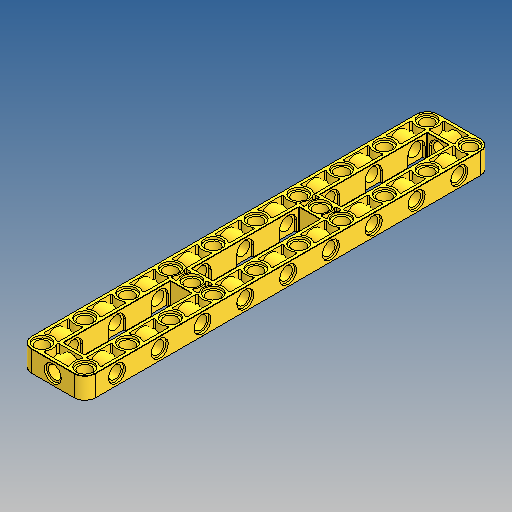
# Autodesk Inventor part: 67491-Yellow
Saved by Autodesk Inventor 2025 (Build 290162010, 162A)
## iProperties
Created: 2012-03-21
Part Number: 67491-Yellow
Document SubType Name: Modeling
Designer: h.muther
Density: 1.06 g/cm^3
Material: ABS Plastic
Mass: 5.69641 g
Surface Area: 80.0064 cm^2
Volume: 5.37397 cm^3
Appearance: Yellow
Author: h.muther
Autodesk Inventor part; units mm, degrees
ref_plane "YZ Plane" through (0, 0, 0) normal (1, 0, 0) x (0, 1, 0)
ref_plane "XZ Plane" through (0, 0, 0) normal (0, 1, 0) x (-1, 0, 0)
ref_plane "XY Plane" through (0, 0, 0) normal (0, 0, 1) x (1, 0, 0)
sketch "Sketch1" plane through (0, 0, 0) normal (0, 0, 1) x (1, 0, 0)
  line L0 (4, -24) -> (4, 24)
  line L1 (-4, 24) -> (-4, -24)
  arc A0 (4, 24) -> (2.8284, 26.8284) centre (0, 24) ccw construction
  arc A1 (-4, -24) -> (4, -24) centre (0, -24) ccw
  circle A2 centre (0, 24) radius 3.2
  circle A3 centre (0, 24) radius 2.4
  line L2 (2.8284, 21.1716) -> (2.8284, 10.8284)
  line L3 (-2.8284, 21.1716) -> (-2.8284, 10.8284)
  arc A4 (-2.8284, 21.1716) -> (2.8284, 21.1716) centre (0, 24) ccw
  arc A5 (2.8284, 10.8284) -> (-2.8284, 10.8284) centre (0, 8) ccw
  circle A6 centre (0, 8) radius 3.2
  circle A7 centre (0, 8) radius 2.4
  line L4 (2.8284, 5.1716) -> (2.8284, -5.1716)
  line L5 (-2.8284, 5.1716) -> (-2.8284, -5.1716)
  arc A8 (-2.8284, 5.1716) -> (2.8284, 5.1716) centre (0, 8) ccw
  arc A9 (2.8284, -5.1716) -> (-2.8284, -5.1716) centre (0, -8) ccw
  circle A10 centre (0, -8) radius 3.2
  circle A11 centre (0, -8) radius 2.4
  line L6 (2.8284, -10.8284) -> (2.8284, -21.1716)
  line L7 (-2.8284, -10.8284) -> (-2.8284, -21.1716)
  arc A12 (-2.8284, -10.8284) -> (2.8284, -10.8284) centre (0, -8) ccw
  arc A13 (2.8284, -21.1716) -> (-2.8284, -21.1716) centre (0, -24) ccw
  circle A14 centre (0, -24) radius 3.2
  circle A15 centre (0, -24) radius 2.4
  line L8 (0, 24) -> (-2.8284, 21.1716) construction
  line L9 (-4, 24) -> (-4, 40)
  line L10 (4, 40) -> (4, 24)
  arc A16 (-2.4, 40) -> (2.4, 40) centre (0, 40) ccw
  arc A17 (-3.2, 40) -> (3.2, 40) centre (0, 40) ccw
  line L11 (-4, 40) -> (-2.4, 40)
  line L12 (2.4, 40) -> (4, 40)
  line L13 (-2.8284, 37.1716) -> (-2.8284, 26.8284)
  arc A18 (2.8284, 26.8284) -> (-2.8284, 26.8284) centre (0, 24) ccw
  arc A19 (-2.8284, 37.1716) -> (2.8284, 37.1716) centre (0, 40) ccw
  line L14 (2.8284, 37.1716) -> (2.8284, 26.8284)
  arc A20 (-2.8284, 26.8284) -> (-4, 24) centre (0, 24) ccw construction
  arc A21 (2.8284, 26.8284) -> (-2.8284, 26.8284) centre (0, 24) ccw
  arc A22 (2.4, 40) -> (-2.4, 40) centre (0, 40) ccw
  arc A23 (3.2, 40) -> (-3.2, 40) centre (0, 40) ccw
  line L15 (-4, 40) -> (-4, 48)
  line L16 (-4, 48) -> (4, 48)
  line L17 (4, 48) -> (4, 40)
  line L18 (-2.8284, 48) -> (-2.8284, 42.8284)
  line L19 (2.8284, 48) -> (2.8284, 42.8284)
  arc A24 (2.8284, 42.8284) -> (-2.8284, 42.8284) centre (0, 40) ccw
  point P0 (0, 0)
  point P1 (-4, 0)
  dimension "d48" = 48
  dimension "d49" = 6.4
  dimension "d50" = 4.8
  dimension "d51" = 16
  dimension "d64" = 16
  dimension "d116" = 45
  dimension "d117" = 56
  dimension "d118" = 8
  dimension "d119" = 16
  dimension "d134" = 8
  constraints: 40 end point, 34 point on circle, 25 centre point, 10 coincident, 9 equal radius, 9 tangent, 7 collinear, 7 vertical, 5 perpendicular, 3 concentric, 3 horizontal alignment, 3 midpoint, 3 point on line, 2 parallel, 2 vertical alignment, 28 other
  measures "d48" distance of A1.centre A0.centre
  measures "d49" diameter of A2
  measures "d50" diameter of A3
  measures "d51" distance of A0.centre A5.centre
  measures "d64" distance of L3.start L5.start
  measures "d116" angle of L8 L1
  measures "d118" diameter of A0
  measures "d119" distance of A16.centre A3.centre
  measures "d134" distance from line of A23.centre L16
extrude "Extrusion1" add sketch "Sketch1" along normal mid plane 8 contours A1 L1 L9 L11 A17 L12 L10 L0 | L12 A23 L11 L15 L16 L18 A24 L19 L17 | A17 L11 A16 L12 | L12 A22 L11 A23 | L19 A24 L18 L16 | A2 | L2 A5 L3 A4 | A6 | L4 A9 L5 A8 | A10 | L6 A13 L7 A12 | A14 | A19 L14 A18 L13
sketch "Sketch6" plane through (0, 0, 4) normal (0, 0, 1) x (1, 0, 0)
  circle A0 centre (0, 24) radius 2.4 projected
  circle A1 centre (0, 24) radius 3.2 projected
  line L0 (2.8284, 21.1716) -> (2.8284, 10.8284) projected
  arc A2 (-2.8284, 21.1716) -> (2.8284, 21.1716) centre (0, 24) ccw projected
  arc A3 (2.8284, 10.8284) -> (-2.8284, 10.8284) centre (0, 8) ccw projected
  line L1 (-2.8284, 21.1716) -> (-2.8284, 10.8284) projected
  circle A4 centre (0, 8) radius 3.2 projected
  line L2 (4, 48) -> (4, -24) projected
  line L3 (4, -24) -> (4, 48) projected
  arc A5 (-2.8284, 5.1716) -> (2.8284, 5.1716) centre (0, 8) ccw projected
  line L4 (2.8284, 5.1716) -> (2.8284, -5.1716) projected
  arc A6 (2.8284, -5.1716) -> (-2.8284, -5.1716) centre (0, -8) ccw projected
  line L5 (-2.8284, 5.1716) -> (-2.8284, -5.1716) projected
  circle A7 centre (0, -8) radius 3.2 projected
  line L6 (2.8284, -10.8284) -> (2.8284, -21.1716) projected
  arc A8 (-2.8284, -10.8284) -> (2.8284, -10.8284) centre (0, -8) ccw projected
  line L7 (-2.8284, -10.8284) -> (-2.8284, -21.1716) projected
  arc A9 (2.8284, -21.1716) -> (-2.8284, -21.1716) centre (0, -24) ccw projected
  circle A10 centre (0, -24) radius 3.2 projected
  line L8 (-2.8284, 37.1716) -> (-2.8284, 26.8284) projected
  arc A11 (-3.2, 40) -> (3.2, 40) centre (0, 40) ccw projected
  arc A12 (-2.8284, 37.1716) -> (2.8284, 37.1716) centre (0, 40) ccw projected
  line L9 (2.8284, 37.1716) -> (2.8284, 26.8284) projected
  arc A13 (2.8284, 26.8284) -> (-2.8284, 26.8284) centre (0, 24) ccw projected
  circle A14 centre (0, 40) radius 2.4 projected
  line L10 (2.8284, 48) -> (2.8284, 42.8284) projected
  arc A15 (2.8284, 42.8284) -> (-2.8284, 42.8284) centre (0, 40) ccw projected
  line L11 (-2.8284, 48) -> (-2.8284, 42.8284) projected
  line L12 (-4, 48) -> (4, 48) projected
  arc A16 (3.2, 40) -> (-3.2, 40) centre (0, 40) ccw projected
  point P0 (-2.4, 40)
  constraints: 1 horizontal alignment
extrude "Extrusion7" cut sketch "Sketch6" against normal blind 0.8 contours A0 | A1 | A4 | A7 | A10 | A16 A11 | A14
extrude "Extrusion8" cut sketch "Sketch6" against normal blind 3.1 contours L0 A3 L1 A2 | A5 L4 A6 L5 | L6 A9 L7 A8 | A12 L9 A13 L8 | L10 A15 L11 L12
sketch "Sketch15" plane through (0, 0, -4) normal (0, 0, -1) x (-1, 0, 0)
  circle A0 centre (0, -8) radius 2.4 projected
  circle A1 centre (0, 8) radius 2.4 projected
  line L0 (-4, -24) -> (-4, 48) projected
  arc A2 (-4, -24) -> (4, -24) centre (0, -24) ccw projected
  line L1 (4, 48) -> (4, -24) projected
  line L2 (-2.8284, -5.1716) -> (-2.8284, 5.1716)
  arc A3 (2.4, -4.8) -> (-2.8284, -5.1716) centre (0, -8) ccw
  arc A4 (-2.8284, 5.1716) -> (2.4, 4.8) centre (0, 8) ccw
  line L3 (2.4, 4.8) -> (2.4, -4.8)
  line L4 (0, -8) -> (-2.8284, -5.1716) construction
  line L5 (-2.8284, -21.1716) -> (-2.8284, -10.8284)
  line L6 (2.4, -20.8) -> (2.4, -11.2)
  arc A5 (2.4, -20.8) -> (-2.8284, -21.1716) centre (0, -24) ccw
  arc A6 (-2.8284, -10.8284) -> (2.4, -11.2) centre (0, -8) ccw
  line L7 (-2.8284, 10.8284) -> (-2.8284, 21.1716)
  line L8 (2.4, 11.2) -> (2.4, 20.8)
  arc A7 (2.4, 11.2) -> (-2.8284, 10.8284) centre (0, 8) ccw
  arc A8 (-2.8284, 21.1716) -> (2.4, 20.8) centre (0, 24) ccw
  circle A9 centre (0, 24) radius 2.4 projected
  circle A10 centre (0, 40) radius 2.4 projected
  line L9 (-2.8284, 26.8284) -> (-2.8284, 37.1716)
  line L10 (2.4, 27.2) -> (2.4, 36.8)
  arc A11 (2.4, 27.2) -> (-2.8284, 26.8284) centre (0, 24) ccw
  arc A12 (-2.8284, 37.1716) -> (2.4, 36.8) centre (0, 40) ccw
  line L11 (-4, 48) -> (4, 48) projected
  line L12 (-2.8284, 48) -> (-2.8284, 42.8284) projected
  arc A13 (2.8284, 42.8284) -> (-2.8284, 42.8284) centre (0, 40) ccw projected
  line L13 (2.4, 43.2) -> (2.4, 48)
  point P0 (0, 0)
  dimension "d109" = 45
  dimension "d111" = 1.6
  constraints: 20 end point, 17 point on circle, 8 centre point, 8 equal radius, 6 coincident, 6 parallel, 4 vertical alignment, 3 collinear, 3 vertical, 2 concentric, 1 perpendicular, 1 point on line
  measures "d109" angle of L0 L4
  measures "d111" distance between parallel lines of L1 L6
extrude "Extrusion19" cut sketch "Sketch15" against normal blind 3.1 contours L11 L13 A13 L12 | L2 A4 L3 A3 | L5 A6 L6 A5 | L7 A8 L8 A7 | L9 A12 L10 A11
mirror "Mirror5" about plane through (0, 0, 0) normal (0, 0, 1) of "Extrusion7"
sketch "Sketch7" plane through (0, 0, 0) normal (1, 0, 0) x (0, 1, 0)
  circle A0 centre (-16, 0) radius 3.6
  circle A1 centre (-16, 0) radius 2.4
  circle A2 centre (0, 0) radius 3.6
  circle A3 centre (0, 0) radius 2.4
  circle A4 centre (16, 0) radius 3.6
  circle A5 centre (16, 0) radius 2.4
  line L0 (-16, 0) -> (0, 0) construction
  line L1 (0, 0) -> (16, 0) construction
  circle A6 centre (32, 0) radius 3.6
  circle A7 centre (32, 0) radius 2.4
  line L2 (48, -4) -> (48, 4) projected
  arc A8 (48, 2.4) -> (48, -2.4) centre (48, 0) ccw
  arc A9 (48, 3.6) -> (48, -3.6) centre (48, 0) ccw
  dimension "d69" = 7.2
  dimension "d70" = 4.8
  dimension "d114" = 16
  dimension "d120" = 16
  constraints: 10 centre point, 8 equal radius, 6 coincident, 5 point on line, 4 end point, 4 point on circle, 2 collinear, 1 horizontal alignment, 1 midpoint
  measures "d69" diameter of A0
  measures "d70" diameter of A1
  measures "d114" distance of L0.start L0.end
  measures "d120" distance of A7.centre L1.end
extrude "Extrusion9" add sketch "Sketch7" against normal up to surface (8 mm away) from surface at 4
extrude "Extrusion10" cut sketch "Sketch7" along normal through all both and the other way through all contours A1 | A3 | A5 | A7 | A8 L2
sketch "Sketch8" plane through (4, -24, 4) normal (1, 0, 0) x (0, 0, -1)
  circle A0 centre (4, 24) radius 2.4 projected
  circle A1 centre (4, 8) radius 2.4 projected
  circle A2 centre (4, 40) radius 2.4 projected
  circle A3 centre (4, 8) radius 3.2
  circle A4 centre (4, 24) radius 3.2
  circle A5 centre (4, 40) radius 3.2
  circle A6 centre (4, 56) radius 2.4 projected
  circle A7 centre (4, 56) radius 3.2
  arc A8 (1.6, 72) -> (6.4, 72) centre (4, 72) ccw projected
  line L0 (0, 72) -> (1.6, 72) projected
  line L1 (6.4, 72) -> (8, 72) projected
  arc A9 (0.8, 72) -> (7.2, 72) centre (4, 72) ccw
  dimension "d75" = 6.4
  constraints: 5 centre point, 4 coincident, 4 equal radius, 2 midpoint, 2 point on circle, 1 concentric
  measures "d75" diameter of A3
extrude "Extrusion11" cut sketch "Sketch8" against normal blind 0.8
sketch "Sketch14" plane through (-4, -24, 4) normal (-1, 0, 0) x (0, 0, 1)
  circle A0 centre (-4, 24) radius 2.4 projected
  circle A1 centre (-4, 8) radius 2.4 projected
  circle A2 centre (-4, 40) radius 2.4 projected
  line L0 (-8, 72) -> (-8, 0) projected
  line L1 (-8, 0) -> (0, 0) projected
  line L2 (-8, 43.2) -> (-4, 43.2)
  arc A3 (-4, 36.8) -> (-4, 43.2) centre (-4, 40) ccw
  line L3 (-4, 36.8) -> (-8, 36.8)
  line L4 (-8, 27.2) -> (-4, 27.2)
  arc A4 (-4, 20.8) -> (-4, 27.2) centre (-4, 24) ccw
  line L5 (-4, 20.8) -> (-8, 20.8)
  line L6 (-8, 11.2) -> (-4, 11.2)
  arc A5 (-4, 4.8) -> (-4, 11.2) centre (-4, 8) ccw
  line L7 (-4, 4.8) -> (-8, 4.8)
  circle A6 centre (-4, 56) radius 2.4 projected
  line L8 (-4, 56) -> (-8, 56) construction
  line L9 (-4, 59.2) -> (-8, 59.2)
  line L10 (-8, 52.8) -> (-4, 52.8)
  arc A7 (-4, 52.8) -> (-4, 59.2) centre (-4, 56) ccw
  line L11 (-8, 52.8) -> (-8, 59.2)
  arc A8 (-6.4, 72) -> (-1.6, 72) centre (-4, 72) ccw projected
  line L12 (-1.6, 72) -> (0, 72) projected
  line L13 (-8, 68.8) -> (-4, 68.8)
  arc A9 (-4, 68.8) -> (-0.8, 72) centre (-4, 72) ccw
  line L14 (-8, 68.8) -> (-8, 72)
  line L15 (-8, 72) -> (-0.8, 72)
  line L16 (0, 72) -> (-1.6, 72) projected
  point P0 (-8, 48)
  point P1 (-8, 64)
  point P2 (-6, 56)
  dimension "d106" = 6.4
  constraints: 28 end point, 10 point on circle, 9 tangent, 6 horizontal, 5 centre point, 4 concentric, 4 equal radius, 4 parallel, 2 midpoint, 1 collinear, 1 perpendicular, 1 vertical, 9 other
  measures "d106" diameter of A3
extrude "Extrusion18" cut sketch "Sketch14" against normal blind 0.8 contours L15 A8 L12 A9 L13 L0 | L9 A7 L10 L0 | L2 A3 L3 L0 | L4 A4 L5 L0 | L6 A5 L7 L0
sketch "Skizze16" plane through (0, 0, -4) normal (0, 0, -1) x (-1, 0, 0)
  arc A0 (-4, -24) -> (4, -24) centre (0, -24) ccw projected
  line L0 (4, -19.2) -> (4, -24) projected
  arc A1 (2.4, -20.8) -> (-2.8284, -21.1716) centre (0, -24) ccw projected
  line L1 (0, -28) -> (8, -28)
  line L2 (8, -28) -> (8, -20)
  line L3 (8, -20) -> (4, -20)
  line L4 (4, 28.8) -> (4, 19.2) projected
  line L5 (8, 28) -> (4, 28)
  line L6 (4, 28) -> (4, 20)
  line L7 (4, 20) -> (8, 20)
  line L8 (8, 20) -> (8, 28)
  circle A2 centre (8, 24) radius 2.4
  circle A3 centre (0, 24) radius 2.4 projected
  point P0 (0, 0)
  point P1 (4, 24)
  point P2 (8, 21.6)
  point P3 (8, 26.4)
  point P4 (4, 28)
  dimension "d121" = 8
  constraints: 14 end point, 3 midpoint, 3 perpendicular, 2 collinear, 2 horizontal, 2 parallel, 1 centre point, 1 equal radius, 1 point on circle, 1 point on line, 1 tangent
  measures "d121" distance from line of A0.centre L2
extrude "Extrusion20" add sketch "Skizze16" against normal up to surface (8 mm away) contours A0 L0 L3 L2 L1 | L5 L8 A2 L7 L4
sketch "Skizze20" plane through (0, 0, -4) normal (0, 0, -1) x (-1, 0, 0)
  arc A0 (8, 26.4) -> (8, 21.6) centre (8, 24) ccw projected
  circle A1 centre (0, 24) radius 3.2 projected
  circle A2 centre (8, 24) radius 3.2
  point P0 (0, 0)
  constraints: 1 centre point, 1 coincident, 1 equal radius
extrude "Extrusion27" cut sketch "Skizze20" against normal up to surface (0.8 mm away) contours A2
sketch "Skizze21" plane through (0, 0, 4) normal (0, 0, 1) x (1, 0, 0)
  arc A0 (-8, 21.6) -> (-8, 26.4) centre (-8, 24) ccw projected
  circle A1 centre (0, 24) radius 3.2 projected
  circle A2 centre (-8, 24) radius 3.2
  point P0 (0, 0)
  constraints: 1 centre point, 1 coincident, 1 equal radius
extrude "Extrusion28" cut sketch "Skizze21" against normal up to surface (0.8 mm away) contours A2
sketch "Skizze17" plane through (0, 0, -4) normal (0, 0, -1) x (-1, 0, 0)
  line L0 (0, -28) -> (8, -28) projected
  line L1 (8, -28) -> (8, -20) projected
  line L2 (8, -20) -> (4, -20) projected
  circle A0 centre (0, -24) radius 3.2 projected
  arc A1 (2.4, -20.8) -> (-2.8284, -21.1716) centre (0, -24) ccw projected
  line L3 (8, -26.828) -> (2.8289, -26.828)
  arc A2 (2.8289, -26.828) -> (3.2, -21.6) centre (0, -24) ccw
  line L4 (3.2, -21.6) -> (8, -21.6)
  arc A3 (8, 27.2) -> (8, 20.8) centre (8, 24) ccw projected
  line L5 (8, 28) -> (4, 28) projected
  line L6 (4, 20) -> (8, 20) projected
  circle A4 centre (0, 24) radius 3.2 projected
  line L7 (3.3038, 21.172) -> (4.6962, 21.172)
  line L8 (3.3038, 26.828) -> (4.6962, 26.828)
  arc A5 (2.9814, 21.8089) -> (2.9814, 26.1911) centre (0, 24) ccw
  arc A6 (5.0186, 26.1911) -> (5.0186, 21.8089) centre (8, 24) ccw
  arc A7 (5.0186, 26.1911) -> (4.6962, 26.828) centre (4.6962, 26.428) ccw
  arc A8 (4.6962, 21.172) -> (5.0186, 21.8089) centre (4.6962, 21.572) ccw
  arc A9 (2.9814, 21.8089) -> (3.3038, 21.172) centre (3.3038, 21.572) ccw
  arc A10 (3.3038, 26.828) -> (2.9814, 26.1911) centre (3.3038, 26.428) ccw
  point P0 (0, 0)
  point P1 (2.3859, 21.172)
  point P2 (5.6141, 21.172)
  point P3 (2.3859, 26.828)
  point P4 (5.6141, 26.828)
  point P5 (6, 20)
  point P6 (4.3, 24)
  point P7 (3.7, 24)
  dimension "d124" = 1.6
  dimension "d125" = 1.172
  dimension "d150" = 1.172
  dimension "d151" = 1.172
  dimension "d152" = 0.6
  dimension "d153" = 0.4
  constraints: 20 point on circle, 8 end point, 8 tangent, 7 centre point, 6 point on line, 5 equal radius, 3 concentric, 3 horizontal, 1 midpoint, 1 perpendicular
  measures "d124" distance between parallel lines of L2 L4
  measures "d125" distance between parallel lines of L0 L3
  measures "d150" distance from line of point (6, 20) L7
  measures "d151" distance between parallel lines of L8 L5
  measures "d152" distance of point (4.3, 24) point (3.7, 24)
  measures "d153" radius of A7
extrude "Extrusion21" cut sketch "Skizze17" against normal up to surface (3.1 mm away) contours L3 A2 L4 L1 | A9 A5 A10 L8 A7 A6 A8 L7
sketch "Skizze18" plane through (0, 0, 4) normal (0, 0, 1) x (1, 0, 0)
  arc A0 (2.8284, -21.1716) -> (-2.8284, -21.1716) centre (0, -24) ccw projected
  line L0 (-8, -20) -> (-4, -20) projected
  line L1 (-8, -28) -> (-8, -20) projected
  circle A1 centre (0, -24) radius 3.2 projected
  line L2 (-8, -26.828) -> (-2.8289, -26.828) projected
  line L3 (-8, -26.828) -> (-3.6694, -26.828)
  arc A2 (-3.3359, -21.7927) -> (-3.3359, -26.2073) centre (0, -24) ccw
  line L4 (-8, -21.172) -> (-3.6694, -21.172)
  arc A3 (-3.3359, -21.7927) -> (-3.6694, -21.172) centre (-3.6694, -21.572) ccw
  arc A4 (-3.6694, -26.828) -> (-3.3359, -26.2073) centre (-3.6694, -26.428) ccw
  arc A5 (-5.0186, 21.8089) -> (-5.0186, 26.1911) centre (-8, 24) ccw projected
  arc A6 (-4.6962, 26.828) -> (-5.0186, 26.1911) centre (-4.6962, 26.428) ccw projected
  line L5 (-3.3038, 26.828) -> (-4.6962, 26.828) projected
  arc A7 (-2.9814, 26.1911) -> (-3.3038, 26.828) centre (-3.3038, 26.428) ccw projected
  arc A8 (-2.9814, 26.1911) -> (-2.9814, 21.8089) centre (0, 24) ccw projected
  arc A9 (-3.3038, 21.172) -> (-2.9814, 21.8089) centre (-3.3038, 21.572) ccw projected
  line L6 (-4.6962, 21.172) -> (-3.3038, 21.172) projected
  arc A10 (-5.0186, 21.8089) -> (-4.6962, 21.172) centre (-4.6962, 21.572) ccw projected
  point P0 (0, 0)
  point P1 (-2.8289, -21.172)
  dimension "d128" = 1.172
  dimension "d129" = 0.4
  constraints: 8 point on circle, 4 end point, 4 point on line, 4 tangent, 3 centre point, 2 equal radius, 1 collinear, 1 concentric, 1 horizontal
  measures "d128" distance between parallel lines of L0 L4
  measures "d129" radius of A3
extrude "Extrusion22" cut sketch "Skizze18" against normal up to surface (3.1 mm away) contours L1 L4 A3 A2 A4 L2 | A5 A6 L5 A7 A8 A9 L6 A10
sketch "Skizze19" plane through (-8, -20, -4) normal (0, 1, 0) x (1, 0, 0)
  line L0 (0, 0) -> (4, 0) projected
  line L1 (0, 0) -> (0, -8) projected
  line L2 (3.2, 0) -> (3.2, -4)
  line L3 (0, -4.9) -> (4.3306, -4.9) projected
  arc A0 (0, -7.2) -> (3.2, -4) centre (0, -4) ccw
  line L4 (0, -7.2) -> (0, 0)
  line L5 (0, 0) -> (3.2, 0)
  point P0 (8, -4)
  point P1 (0, -7.2)
  dimension "d135" = 3.2
  constraints: 6 end point, 2 perpendicular, 2 point on circle, 1 centre point, 1 collinear, 1 midpoint, 1 parallel, 1 point on line, 1 tangent
  measures "d135" radius of A0
extrude "Extrusion23" cut sketch "Skizze19" against normal blind 0.8
fillet "Fillet2" radius 0.4 38 edges at (-2.8284, 21.1716, 2.45) (-2.8284, 10.8284, 2.45) (2.8284, 10.8284, 2.45) (2.8284, 21.1716, 2.45) (-2.8284, -21.1716, 2.45) (-2.8284, -10.8284, 2.45) (2.8284, -10.8284, 2.45) (2.8284, -21.1716, 2.45) (2.8284, -5.1716, 2.45) (-2.8284, -5.1716, 2.45) (-2.8284, 5.1716, 2.45) (2.8284, 5.1716, 2.45) (-2.4, 20.8, -2.45) (2.8284, 21.1716, -2.45) (2.8284, 10.8284, -2.45) (-2.4, 11.2, -2.45) (-2.4, 4.8, -2.45) (2.8284, 5.1716, -2.45) (-2.4, -4.8, -2.45) (2.8284, -5.1716, -2.45) (-2.4, -11.2, -2.45) (2.8284, -10.8284, -2.45) (2.8284, -21.1716, -2.45) (-2.4, -20.8, -2.45) (-3.2, -21.6, -2.45) (-2.8289, -26.828, -2.45) (-2.8284, 42.8284, 2.45) (2.8284, 42.8284, 2.45) (2.8284, 26.8284, 2.45) (-2.8284, 26.8284, 2.45) (-2.8284, 37.1716, 2.45) (2.8284, 37.1716, 2.45) (-2.4, 43.2, -2.45) (2.8284, 42.8284, -2.45) (2.8284, 37.1716, -2.45) (-2.4, 36.8, -2.45) (-2.4, 27.2, -2.45) (2.8284, 26.8284, -2.45)
fillet "Fillet2" radius 0.1 20 edges at (-4, 38, 4) (-4, 0, 4) (4, 12, 4) (2.8284, -26.8284, 4) (-4, 8, -4) (-4, -8, -4) (-4, -19.6, -4) (-4, 40, -4) (-4, 19.6, -4) (-4, 28.4, -4) (2.8284, -26.8284, -4) (4, 12, -4) (-6, -20, 4) (-4.4, -20, -4) (-4, -20, 0) (-4, 28, 0) (-6, 28, 4) (-6, 20, 4) (-6, 28, -4) (-6, 20, -4)
sketch "Sketch12" plane through (-4, -28, 2.9) normal (0, -1, 0) x (1, 0, 0)
  line L0 (-4, -6.8) -> (-4, 1) projected
  circle A0 centre (-4, -2.9) radius 2.4
  circle A1 centre (-4, -2.9) radius 3.6
  circle A2 centre (-4, -2.9) radius 3.2
  point P0 (-4, 0.3)
  point P1 (-4, -6.1)
  point P2 (-4, -0.5)
  point P3 (-4, -5.3)
  dimension "d133" = 6.4
  dimension "d138" = 7.2
  dimension "d139" = 4.8
  constraints: 3 centre point, 2 coincident, 1 midpoint
  measures "d133" diameter of A2
  measures "d138" diameter of A1
  measures "d139" diameter of A0
extrude "Extrusion24" add sketch "Sketch12" against normal up to surface (7.2 mm away) contours L0 A0 A2 | L0 A0 picked at (-1.1135, -2.4846) picked at (-3.042, -3.0981)
extrude "Extrusion25" cut sketch "Sketch12" against normal up to surface (7.2 mm away) contours L0 A0 picked at (-3.042, -3.0981)
extrude "Extrusion26" cut sketch "Sketch12" against normal blind 0.8 contours L0 A0 A2 picked at (-1.1135, -2.4846)
mirror "Mirror4" about plane through (-4, 48, 0) normal (0, 1, 0)
mirror "Mirror3" about plane through (-8, -20, -4) normal (-1, 0, 0)
equation "\"lf\" = 0.1"
equation "\"tf\" = 0.4"
body "Solid1"
